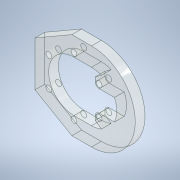
# Autodesk Inventor part: Standalone_Valve_Spacer_Plate
Saved by Autodesk Inventor 2020 (Build 240168000, 168)
## iProperties
Created: 2021-07-01
Part Number: Standalone_Valve_Spacer_Plate
Material: Glass
Document SubType Name: Modeling
Designer: Workshop
Density: 2.18 g/cm^3
Appearance: Clear
Author: Workshop
Autodesk Inventor part; units mm, degrees
ref_plane "YZ Plane" through (0, 0, 0) normal (1, 0, 0) x (0, 1, 0)
ref_plane "XZ Plane" through (0, 0, 0) normal (0, 1, 0) x (-1, 0, 0)
ref_plane "XY Plane" through (0, 0, 0) normal (0, 0, 1) x (1, 0, 0)
sketch "Sketch1" plane through (0, 0, 0) normal (0, 0, 1) x (1, 0, 0)
  arc A0 (8.9957, -22.4752) -> (8.9947, 22.4772) centre (8.9954, 0.001) ccw projected
  line L0 (8.9947, 22.4772) -> (-1.0767, 22.4739) projected
  line L1 (-1.0767, 22.4739) -> (-20.0043, 11.546) projected
  line L2 (-20.0043, 11.546) -> (-20.0043, -11.548) projected
  line L3 (-20.0043, -11.548) -> (-1.0759, -22.4763) projected
  line L4 (-1.0759, -22.4763) -> (8.9957, -22.4752) projected
  arc A1 (8.9954, -13) -> (14.0866, -11.9616) centre (8.9954, 0) ccw projected
  line L5 (14.0866, -11.9616) -> (10.9211, -9.6812) projected
  line L6 (10.9211, -9.6812) -> (10.9211, -7.4615) projected
  arc A2 (12.9211, -5.4615) -> (10.9211, -7.4615) centre (12.9211, -7.4615) ccw projected
  line L7 (12.9211, -5.4615) -> (20.7926, -5.4615) projected
  arc A3 (20.7926, -5.4615) -> (20.7926, 5.4615) centre (8.9954, 0) ccw projected
  line L8 (20.7926, 5.4615) -> (12.9211, 5.4615) projected
  arc A4 (10.9211, 7.4615) -> (12.9211, 5.4615) centre (12.9211, 7.4615) ccw projected
  line L9 (10.9211, 7.4615) -> (10.9211, 9.6812) projected
  line L10 (10.9211, 9.6812) -> (14.0866, 11.9616) projected
  arc A5 (14.0866, 11.9616) -> (8.9955, 13) centre (8.9954, 0) ccw projected
  line L11 (8.9955, 13) -> (-0.0043, 13) projected
  arc A6 (-0.0043, 13) -> (-0.0043, -13) centre (-0.0043, 0) ccw projected
  line L12 (-0.0043, -13) -> (8.9954, -13) projected
  circle A7 centre (12.9211, -7.4615) radius 1.5 projected
  circle A8 centre (12.9211, 7.4615) radius 1.5 projected
  circle A9 centre (-0.0043, -14.929) radius 1.5 projected
  circle A10 centre (-12.9298, -7.4665) radius 1.5 projected
  circle A11 centre (-12.9298, 7.4585) radius 1.5 projected
  circle A12 centre (-0.0043, 14.921) radius 1.5 projected
  circle A13 centre (-0.0043, -14.929) radius 1.5 projected
  circle A14 centre (-12.9298, -7.4665) radius 1.5 projected
  circle A15 centre (-12.9298, 7.4585) radius 1.5 projected
  circle A16 centre (-0.0043, 14.921) radius 1.5 projected
  point P0 (0, 0)
extrude "Extrusion1" add sketch "Sketch1" along normal mid plane 5
body "Solid1"
